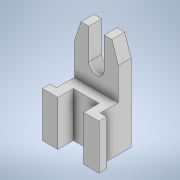
# Autodesk Inventor part: 6
Saved by Autodesk Inventor 2022 (Build 260153000, 153)
## iProperties
Created: 2022-03-14
Part Number: 6
Material: Všeobecné
Document SubType Name: Modeling
Designer: Šimon
Density: 1 g/cm^3
Appearance: Výchozí
Author: Šimon
Autodesk Inventor part; units mm, degrees
ref_plane "YZ Plane" through (0, 0, 0) normal (1, 0, 0) x (0, 1, 0)
ref_plane "XZ Plane" through (0, 0, 0) normal (0, 1, 0) x (-1, 0, 0)
ref_plane "XY Plane" through (0, 0, 0) normal (0, 0, 1) x (1, 0, 0)
sketch "Náčrt1" plane through (0, 0, 0) normal (0, 0, 1) x (1, 0, 0)
  line L0 (0, 0) -> (0, 60)
  line L1 (5, 75) -> (0, 60)
  line L2 (5, 75) -> (11, 75)
  line L3 (11, 75) -> (11, 51)
  arc A0 (11, 51) -> (23, 51) centre (17, 51) ccw
  line L4 (23, 51) -> (23, 75)
  line L5 (23, 75) -> (29, 75)
  line L6 (34, 60) -> (29, 75)
  line L7 (34, 60) -> (34, 0)
  line L8 (34, 0) -> (0, 0)
  dimension "d0" = 60
  dimension "d3" = 6
  dimension "d4" = 24
  dimension "d5" = 12
  dimension "d6" = 6
  constraints: 18 end point, 3 perpendicular, 3 vertical, 2 point on circle, 1 centre point, 1 horizontal, 1 tangent
  measures "d0" distance of L0.start L0.end
  measures "d3" distance of L1.start L2.end
  measures "d4" distance of L2.end L3.end
  measures "d5" distance of L3.end L4.start
  measures "d6" distance of L4.end L5.end
extrude "Vysunutí1" add sketch "Náčrt1" along normal blind 10
sketch "Náčrt2" plane through (0, 0, 0) normal (0, -1, 0) x (1, 0, 0)
  line L0 (5, 10) -> (0, 10) projected
  line L1 (34, 0) -> (34, 10) projected
  line L2 (0, 10) -> (34, 10)
  line L3 (34, 10) -> (34, 24)
  line L4 (34, 24) -> (39, 24)
  line L5 (39, 24) -> (39, 30)
  line L6 (-5, 30) -> (-5, 24)
  line L7 (-5, 24) -> (0, 24)
  line L8 (0, 24) -> (0, 10)
  line L9 (-5, 30) -> (7, 30)
  line L10 (7, 30) -> (7, 18)
  line L11 (7, 18) -> (27, 18)
  line L12 (27, 18) -> (27, 30)
  line L13 (27, 30) -> (39, 30)
  point P0 (0, 0)
  dimension "d11" = 14
  dimension "d12" = 5
  dimension "d13" = 6
  dimension "d14" = 44
  dimension "d15" = 6
  dimension "d16" = 12
  dimension "d17" = 12
  dimension "d18" = 20
  constraints: 24 end point, 8 perpendicular, 3 point on line, 1 horizontal, 1 vertical
  measures "d11" distance of L1.end L3.end
  measures "d12" distance of L3.end L4.end
  measures "d13" distance of L4.end L5.end
  measures "d14" distance of L5.end L6.start
  measures "d15" distance of L6.start L6.end
  measures "d16" distance of L6.start L9.end
  measures "d17" distance of L9.end L10.end
  measures "d18" distance of L10.end L11.end
extrude "Vysunutí2" add sketch "Náčrt2" against normal blind 35
